Autodesk Fusion 360 part; units mm, degrees
(part 2 of 2)
  line L429 (247.65, -23.8125) -> (247.65, -42.8625)
  line L430 (247.65, -42.8625) -> (219.075, -23.8125) construction
  line L431 (219.075, -42.8625) -> (247.65, -23.8125) construction
  line L432 (223.8375, -61.9125) -> (247.65, -61.9125)
  line L433 (247.65, -61.9125) -> (247.65, -42.8625)
  line L434 (252.4125, -61.9125) -> (252.4125, -23.8125)
  line L435 (252.4125, -23.8125) -> (328.6125, -23.8125)
  line L436 (290.5125, -100.0125) -> (328.6125, -100.0125)
  line L437 (185.7375, -80.9625) -> (42.8625, -80.9625)
  line L438 (23.8125, -100.0125) -> (0, -100.0125)
  line L439 (290.5125, -19.05) -> (328.6125, -19.05)
  line L440 (247.65, -19.05) -> (209.55, -19.05)
  line L441 (219.075, -23.8125) -> (47.625, -23.8125)
  line L442 (47.625, -19.05) -> (85.725, -19.05)
  line L443 (128.5875, -19.05) -> (166.6875, -19.05)
  line L444 (180.975, -104.775) -> (185.7375, -100.0125)
  line L445 (209.55, -104.775) -> (204.7875, -100.0125)
  line L446 (266.7, -104.775) -> (271.4625, -100.0125)
  line L447 (47.625, -104.775) -> (42.8625, -100.0125)
  line L448 (47.625, -104.775) -> (180.975, -104.775)
  line L449 (209.55, -104.775) -> (266.7, -104.775)
  line L450 (-9.525, -109.5375) -> (-9.525, 9.525)
  line L451 (-9.525, 9.525) -> (338.1375, 9.525)
  line L452 (338.1375, -109.5375) -> (338.1375, 9.525)
  line L453 (290.5125, -109.5375) -> (338.1375, -109.5375)
  line L454 (275.4079, -109.5375) -> (290.5125, -109.5375)
  line L455 (270.6454, -114.3) -> (275.4079, -109.5375)
  line L456 (205.6046, -114.3) -> (270.6454, -114.3)
  line L457 (205.6046, -114.3) -> (200.8421, -109.5375)
  line L458 (200.8421, -109.5375) -> (189.6829, -109.5375)
  line L459 (184.9204, -114.3) -> (189.6829, -109.5375)
  line L460 (184.9204, -114.3) -> (43.6796, -114.3)
  line L461 (43.6796, -114.3) -> (38.9171, -109.5375)
  line L462 (38.9171, -109.5375) -> (23.8125, -109.5375)
  line L463 (23.8125, -109.5375) -> (-9.525, -109.5375)
  point P0 (9.525, -9.525)
  point P1 (38.1, -9.525)
  point P2 (38.1, -33.3375)
  point P3 (95.25, -9.525)
  point P4 (119.0625, -9.525)
  point P5 (176.2125, -9.525)
  point P6 (200.025, -9.525)
  point P7 (280.9875, -9.525)
  point P8 (257.175, -9.525)
  point P9 (257.175, -95.25)
  point P10 (238.125, -76.2)
  point P11 (219.075, -95.25)
  point P12 (195.2625, -90.4875)
  point P13 (114.3, -95.25)
  point P14 (33.3375, -90.4875)
  point P15 (280.9875, -90.4875)
  point P16 (261.9375, -71.4375)
  point P17 (209.55, -71.4375)
  point P18 (233.3625, -33.3375)
  dimension "d1" = 19.05
  dimension "d2" = 19.05
  dimension "d3" = 19.05
  dimension "d4" = 19.05
  dimension "d5" = 19.05
  dimension "d6" = 19.05
  dimension "d7" = 19.05
  dimension "d8" = 19.05
  dimension "d9" = 19.05
  dimension "d10" = 19.05
  dimension "d11" = 19.05
  dimension "d12" = 133.35
  dimension "d13" = 19.05
  dimension "d14" = 19.05
  dimension "d15" = 19.05
  dimension "d16" = 19.05
  dimension "d17" = 28.575
  dimension "d18" = 19.05
  dimension "d19" = -9.525
  constraint horizontal L319
  constraint perpendicular L319 L320
  constraint parallel L319 L321
  constraint parallel L320 L322
  constraint coincident L323 P0
  constraint coincident L324 P0
  constraint horizontal L325
  constraint perpendicular L325 L326
  constraint parallel L325 L327
  constraint parallel L326 L328
  constraint coincident L329 P1
  constraint coincident L330 P1
  constraint coincident L313 L325.start
  constraint horizontal L331
  constraint perpendicular L331 L332
  constraint parallel L331 L333
  constraint parallel L332 L334
  constraint coincident L335 P2
  constraint coincident L336 P2
  constraint horizontal L337
  constraint perpendicular L337 L338
  constraint parallel L337 L339
  constraint parallel L338 L340
  constraint coincident L341 P3
  constraint coincident L342 P3
  constraint horizontal L343
  constraint perpendicular L343 L344
  constraint parallel L343 L345
  constraint parallel L344 L346
  constraint coincident L347 P4
  constraint coincident L348 P4
  constraint coincident L313 L343.start
  constraint horizontal L349
  constraint perpendicular L349 L350
  constraint parallel L349 L351
  constraint parallel L350 L352
  constraint coincident L353 P5
  constraint coincident L354 P5
  constraint coincident L313 L349.start
  constraint horizontal L355
  constraint perpendicular L355 L356
  constraint parallel L355 L357
  constraint parallel L356 L358
  constraint coincident L359 P6
  constraint coincident L360 P6
  constraint coincident L313 L355.start
  constraint horizontal L361
  constraint perpendicular L361 L362
  constraint parallel L361 L363
  constraint parallel L362 L364
  constraint coincident L365 P7
  constraint coincident L366 P7
  constraint coincident L313 L361.start
  constraint horizontal L367
  constraint perpendicular L367 L368
  constraint parallel L367 L369
  constraint parallel L368 L370
  constraint coincident L371 P8
  constraint coincident L372 P8
  constraint coincident L313 L367.start
  constraint horizontal L373
  constraint perpendicular L373 L374
  constraint parallel L373 L375
  constraint parallel L374 L376
  constraint coincident L377 P9
  constraint coincident L378 P9
  constraint coincident L373.start L448
  constraint horizontal L379
  constraint perpendicular L379 L380
  constraint parallel L379 L381
  constraint parallel L380 L382
  constraint coincident L383 P10
  constraint coincident L384 P10
  constraint horizontal L385
  constraint perpendicular L385 L386
  constraint parallel L385 L387
  constraint parallel L386 L388
  constraint coincident L389 P11
  constraint coincident L390 P11
  constraint horizontal L391
  constraint perpendicular L391 L392
  constraint parallel L391 L393
  constraint parallel L392 L394
  constraint coincident L395 P12
  constraint coincident L396 P12
  constraint horizontal L397
  constraint perpendicular L397 L398
  constraint parallel L397 L399
  constraint parallel L398 L400
  constraint coincident L401 P13
  constraint coincident L402 P13
  constraint horizontal L403
  constraint coincident L405 P14
  constraint coincident L406 P14
  constraint horizontal L407
  constraint perpendicular L407 L408
  constraint parallel L407 L409
  constraint parallel L408 L410
  constraint coincident L411 P15
  constraint coincident L412 P15
  constraint horizontal L413
  constraint perpendicular L413 L414
  constraint parallel L413 L415
  constraint parallel L414 L416
  constraint coincident L417 P16
  constraint coincident L418 P16
  constraint coincident L301 L419.end
  constraint perpendicular L301 L419
  constraint horizontal L420
  constraint perpendicular L420 L421
  constraint parallel L420 L422
  constraint parallel L421 L423
  constraint coincident L424 P17
  constraint coincident L425 P17
  constraint midpoint L393 L420.start
  constraint horizontal L426
  constraint perpendicular L426 L427
  constraint parallel L426 L428
  constraint parallel L427 L429
  constraint coincident L430 P18
  constraint coincident L431 P18
  constraint perpendicular L421 L432
  constraint perpendicular L426 L433
  constraint perpendicular L428 L434
  constraint coincident L305 L435.end
  constraint perpendicular L305 L435
  constraint perpendicular L305 L436
  constraint perpendicular L404 L437
  constraint perpendicular L301 L438
  constraint coincident L305 L439.end
  constraint perpendicular L305 L439
  constraint perpendicular L358 L440
  constraint perpendicular L427 L441
  constraint perpendicular L340 L442
  constraint perpendicular L350 L443
  constraint parallel L396 L444
  constraint perpendicular L444 L445
  constraint perpendicular L377 L446
  constraint perpendicular L446 L447
  constraint collinear L448 L449
  measures "d1" distance of L326.end L327.end
  measures "d2" distance of L331.end L332.end
  measures "d3" distance of L338.end L339.end
  measures "d4" distance of L344.end L345.end
  measures "d5" distance of L350.end L351.end
  measures "d6" distance of L356.end L357.end
  measures "d7" distance of L362.end L363.end
  measures "d8" distance of L368.end L369.end
  measures "d9" distance of L374.end L375.end
  measures "d10" distance of L392.end L393.end
  measures "d11" distance of L391.end L392.end
  measures "d12" distance of L398.end L399.end
  measures "d13" distance of L405.end L404.start
  measures "d14" distance of L403.end L405.end
  measures "d15" distance of L408.end L409.end
  measures "d16" distance of L407.end L408.end
  measures "d17" distance of L427.end L428.end
  measures "d18" distance of L426.end L427.end
extrude "Extrude1" add sketch "plate-2023-07-14T19_23_39.336Z" along normal blind 7.8 contours L301 L305 L313 L320 L321 L326 L327 L331 L338 L339 L344 L345 L351 L352 L356 L357 L362 L363 L369 L370 L375 L376 L380 L381 L382 L385 L386 L394 L408 L413 L414 L419 L420 L421 L428 L429 L432 L433 L434 L435 L439 L440 L441 L442 L443 L445 L446 | L392 L398 L399 L400 L404 L437 L444 L447 | L450 L451 L452 L453 L454 L455 L456 L457 L458 L459 L460 L461 L462 L463 in component "for my desk"
component "for my desk" placed x (1, 0, 0) y (0, 1, 0) z (0, 0, 1) at (0, 0, 0)
equation "d12 = ( 19.05 * 7 ) * 1 mm"
equation "d17 = ( 19.05 * 1.5 ) * 1 mm"
